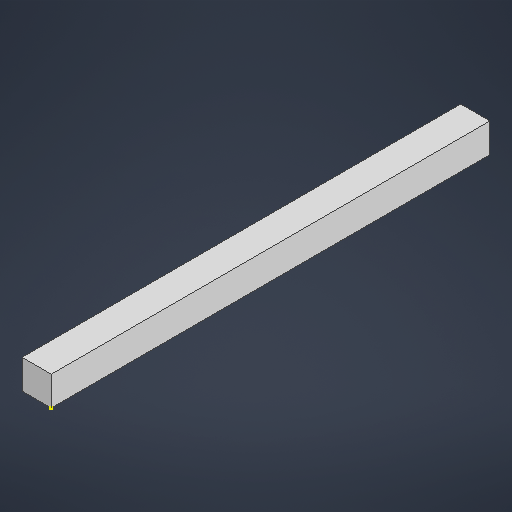
# Autodesk Inventor part: Arm_Pole
Saved by Autodesk Inventor 2026.1 (Build 301233000, 233)
## iProperties
Created: 2025-09-01
Part Number: Arm_Pole
Material: Generic
Document SubType Name: Modeling
Designer: junha
Density: 1 g/cm^3
Appearance: Default
Author: junha
Autodesk Inventor part; units mm, degrees
ref_plane "YZ Plane" through (0, 0, 0) normal (1, 0, 0) x (0, 1, 0)
ref_plane "XZ Plane" through (0, 0, 0) normal (0, 1, 0) x (-1, 0, 0)
ref_plane "XY Plane" through (0, 0, 0) normal (0, 0, 1) x (1, 0, 0)
sketch "Sketch1" plane through (0, 0, 0) normal (0, 1, 0) x (-1, 0, 0)
  line L0 (0, 0) -> (0, -90)
  line L1 (0, -90) -> (10, -90)
  line L2 (10, -90) -> (10, 0)
  line L3 (10, 0) -> (0, 0)
  dimension "d0" = 90
  dimension "d1" = 10
  constraints: 8 end point, 3 perpendicular, 1 vertical
  measures "d0" distance of L0.start L0.end
  measures "d1" distance of L0.end L1.end
extrude "Extrusion1" add sketch "Sketch1" along normal blind 10
sketch "Sketch2" plane through (-10, 0, 0) normal (0, 0, 1) x (1, 0, 0)
  line L0 (0, 0) -> (0, 10) projected
  line L1 (0, 10) -> (10, 10)
  line L2 (10, 10) -> (10, 0)
  line L3 (10, 0) -> (0, 0)
  line L4 (0, 0) -> (0, 10)
  constraints: 8 end point, 2 parallel, 1 horizontal, 1 perpendicular
extrude "Extrusion2" add sketch "Sketch2" along normal blind 60
sketch "Sketch3" plane through (-10, 0, 60) normal (0, 0, 1) x (1, 0, 0)
  point P0 (10, 0)
body "Solid1"
